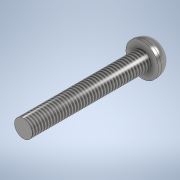
# Autodesk Inventor part: tonrilloM3x20mm
Saved by Autodesk Inventor 2021.5 (Build 255421000, 421)
## iProperties
Created: 2024-11-29
Part Number: tonrilloM3x20mm
Material: Acero inoxidable
Document SubType Name: Modeling
Designer: Joho_
Mass: 1.43784 g
Surface Area: 2.75123 cm^2
Volume: 0.17973 cm^3
Density: 8 g/cm^3
Appearance: Semipulido
Author: Joho_
Autodesk Inventor part; units mm, degrees
ref_plane "YZ Plane" through (0, 0, 0) normal (1, 0, 0) x (0, 1, 0)
ref_plane "XZ Plane" through (0, 0, 0) normal (0, 1, 0) x (-1, 0, 0)
ref_plane "XY Plane" through (0, 0, 0) normal (0, 0, 1) x (1, 0, 0)
sketch "Boceto1" plane through (0, 0, 0) normal (0, 0, 1) x (1, 0, 0)
  circle A0 centre (0, 0) radius 1.5
  circle A1 centre (0, 0) radius 2.75
  dimension "d0" = 3
  dimension "d1" = 5.5
  constraints: 3 coincident, 2 centre point
  measures "d0" diameter of A0
  measures "d1" diameter of A1
extrude "Extrusión1" add sketch "Boceto1" along normal blind 20 contours A0
extrude "Extrusión2" add sketch "Boceto1" against normal blind 2.5 contours A0 | A1
sketch "Boceto2" plane through (0, 0, -2.5) normal (0, 0, -1) x (-1, 0, 0)
  line L0 (1.5, 0) -> (0.75, -1.299)
  line L1 (0.75, -1.299) -> (-0.75, -1.299)
  line L2 (-0.75, -1.299) -> (-1.5, 0)
  line L3 (-1.5, 0) -> (-0.75, 1.299)
  line L4 (-0.75, 1.299) -> (0.75, 1.299)
  line L5 (0.75, 1.299) -> (1.5, 0)
  point P0 (0, 0)
  point P1 (0, 0)
  dimension "d6" = 3
  constraints: 12 end point, 1 coincident, 13 other
  measures "d6" distance of L0.start L2.end
fillet "Empalme1" radius 2 1 edges at (-2.75, 0, -2.5)
extrude "Extrusión4" cut sketch "Boceto2" against normal blind 1.5
thread "Rosca1" size "M3x0.5" class "6g" standard "ANSI Metric M Profile" full length
